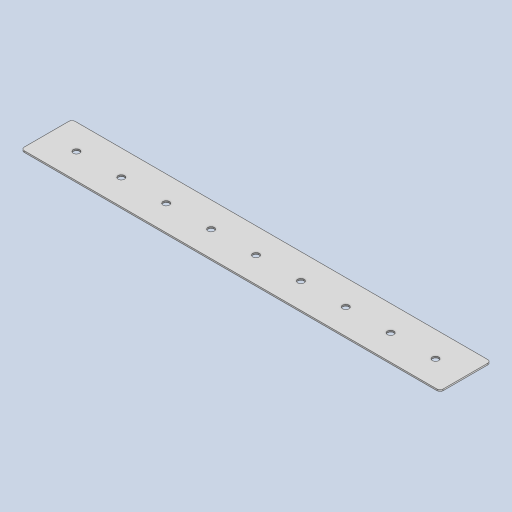
# Autodesk Inventor part: Old-sheet
Saved by Autodesk Inventor 2023 (Build 270158000, 158)
## iProperties
Created: 2024-12-14
Part Number: Old-sheet
Material: Generic
Document SubType Name: Modeling
Designer: kiyo
Density: 1 g/cm^3
Appearance: Default
Author: kiyo
Autodesk Inventor part; units mm, degrees
ref_plane "YZ Plane" through (0, 0, 0) normal (1, 0, 0) x (0, 1, 0)
ref_plane "XZ Plane" through (0, 0, 0) normal (0, 1, 0) x (-1, 0, 0)
ref_plane "XY Plane" through (0, 0, 0) normal (0, 0, 1) x (1, 0, 0)
sketch "スケッチ1" plane through (0, 0, 0) normal (0, 0, 1) x (1, 0, 0)
  line L0 (0, 0) -> (-17, 0)
  line L1 (-17, 0) -> (-17, -140)
  line L2 (-17, -140) -> (0, -140)
  line L3 (0, -140) -> (0, 0)
  circle A0 centre (-8.5, -130) radius 1.1
  circle A1 centre (-8.5, -115) radius 1.1
  circle A2 centre (-8.5, -100) radius 1.1
  circle A3 centre (-8.5, -85) radius 1.1
  circle A4 centre (-8.5, -70) radius 1.1
  circle A5 centre (-8.5, -55) radius 1.1
  circle A6 centre (-8.5, -40) radius 1.1
  circle A7 centre (-8.5, -25) radius 1.1
  circle A8 centre (-8.5, -10) radius 1.1
  dimension "d0" = 140
  dimension "d1" = 17
  dimension "d2" = 2.2
  dimension "d3" = 10
  dimension "d4" = 8.5
  dimension "d7" = 15
  constraints: 9 centre point, 8 end point, 2 parallel, 1 horizontal, 1 perpendicular, 1 vertical, 16 other
  measures "d0" distance of L0.end L1.end
  measures "d1" distance of L1.end L2.end
  measures "d2" diameter of A0
  measures "d3" distance from line of L2 A0.centre
  measures "d4" distance from line of L1 A0.centre
  measures "d7" distance of A0.centre A1.centre
extrude "押し出し1" add sketch "スケッチ1" along normal blind 0.5
fillet "フィレット1" radius 1 4 edges at (-17, -140, 0.25) (0, -140, 0.25) (0, 0, 0.25) (-17, 0, 0.25)
equation "\"d4\" = 0.5 * d1"
